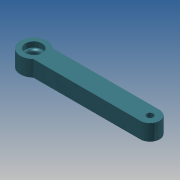
# Autodesk Inventor part: proximal thin arm
Saved by Autodesk Inventor 2013 (Build 170138000, 138)
## iProperties
Created: 2017-03-30
Part Number: proximal thin arm
Material: Generic
Document SubType Name: Modeling
Designer: employee
Density: 1 g/cm^3
Author: employee
Autodesk Inventor part; units mm, degrees
ref_plane "YZ Plane" through (0, 0, 0) normal (1, 0, 0) x (0, 1, 0)
ref_plane "XZ Plane" through (0, 0, 0) normal (0, 1, 0) x (-1, 0, 0)
ref_plane "XY Plane" through (0, 0, 0) normal (0, 0, 1) x (1, 0, 0)
sketch "Sketch1" plane through (0, 0, 0) normal (0, 0, 1) x (1, 0, 0)
  line L0 (0, 12.6) -> (153, 12.6)
  arc A0 (153, -12.6) -> (153, 12.6) centre (153, 0) ccw
  line L1 (153, -12.6) -> (0, -12.6)
  arc A1 (0, 12.6) -> (0, -12.6) centre (0, 0) ccw
  circle A2 centre (0, 0) radius 7.5
  circle A3 centre (153, 0) radius 4.25
  dimension "d0" = 153
  dimension "d2" = 12.6
  dimension "d3" = 15
  dimension "d4" = 8.5
  constraints: 4 centre point, 4 end point, 4 point on circle, 4 tangent, 3 coincident, 1 horizontal, 1 parallel
  measures "d0" distance of L0.start L0.end
  measures "d2" radius of A1
  measures "d3" diameter of A2
  measures "d4" diameter of A3
extrude "Extrusion1" add sketch "Sketch1" along normal blind 21.1
sketch "Sketch2" plane through (0, 0, 21.1) normal (0, 0, 1) x (1, 0, 0)
  circle A0 centre (0, 0) radius 7.5 projected
  arc A1 (0, 12.6) -> (0, -12.6) centre (0, 0) ccw projected
  circle A2 centre (0, 0) radius 11
  dimension "d7" = 22
  constraints: 1 centre point, 1 coincident
  measures "d7" diameter of A2
extrude "Extrusion2" cut sketch "Sketch2" against normal blind 7
sketch "Sketch6" plane through (0, 0, 21.1) normal (0, 0, 1) x (1, 0, 0)
  circle A0 centre (0, 0) radius 11 projected
  arc A1 (0, 12.6) -> (0, -12.6) centre (0, 0) ccw projected
  circle A2 centre (0, 0) radius 17.5
  dimension "d25" = 35
  constraints: 1 centre point, 1 coincident
  measures "d25" diameter of A2
extrude "Extrusion5" add sketch "Sketch6" against normal up to surface (21.1 mm away)
sketch "Sketch7" plane through (0, 0, 0) normal (0, 0, -1) x (-1, 0, 0)
  circle A0 centre (0, 0) radius 7.5 projected
  circle A1 centre (0, 0) radius 11 projected
extrude "Extrusion6" cut sketch "Sketch7" against normal blind 7
sketch "Sketch8" plane through (0, 0, 0) normal (0, 0, -1) x (-1, 0, 0)
  circle A0 centre (-153, 0) radius 4.25 projected
  arc A1 (-153, 12.6) -> (-153, -12.6) centre (-153, 0) ccw projected
  line L0 (-145.4944, 0) -> (-149.2472, -6.5)
  line L1 (-149.2472, -6.5) -> (-156.7528, -6.5)
  line L2 (-156.7528, -6.5) -> (-160.5056, 0)
  line L3 (-160.5056, 0) -> (-156.7528, 6.5)
  line L4 (-156.7528, 6.5) -> (-149.2472, 6.5)
  line L5 (-149.2472, 6.5) -> (-145.4944, 0)
  dimension "d31" = 13
  constraints: 12 end point, 1 coincident, 13 other
  measures "d31" distance between parallel lines of L1 L4
extrude "Extrusion7" cut sketch "Sketch8" against normal blind 8
fillet "Fillet1" radius 3.5 1 edges at (-7.5, 0, 14.1)
fillet "Fillet2" radius 3.5 1 edges at (-7.5, 0, 7)
body "Solid1"
